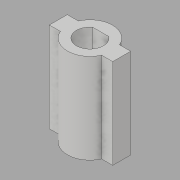
# Autodesk Inventor part: DispenserCoupling
Saved by Autodesk Inventor 2017 (Build 210142000, 142)
## iProperties
Created: 2017-02-22
Part Number: DispenserCoupling
Material: Generic
Document SubType Name: Modeling
Designer: gmarsh
Density: 1 g/cm^3
Appearance: Default
Author: gmarsh
Autodesk Inventor part; units mm, degrees
ref_plane "YZ Plane" through (0, 0, 0) normal (1, 0, 0) x (0, 1, 0)
ref_plane "XZ Plane" through (0, 0, 0) normal (0, 1, 0) x (-1, 0, 0)
ref_plane "XY Plane" through (0, 0, 0) normal (0, 0, 1) x (1, 0, 0)
sketch "Sketch1" plane through (0, 0, 0) normal (0, 0, 1) x (1, 0, 0)
  line L0 (7.0628, 2) -> (7.0628, -2)
  line L1 (-7.0394, -2) -> (-7.0394, 2)
  line L2 (-7.0394, 2) -> (-4.5826, 2)
  line L3 (4.5826, 2) -> (7.0628, 2)
  line L4 (7.0628, -2) -> (4.5826, -2)
  line L5 (-4.5826, -2) -> (-7.0394, -2)
  arc A0 (-4.5826, -2) -> (4.5826, -2) centre (0, 0) ccw
  arc A1 (4.5826, 2) -> (-4.5826, 2) centre (0, 0) ccw
  constraints: 12 end point, 5 parallel, 4 point on circle, 2 centre point, 2 horizontal, 2 perpendicular, 1 coincident
extrude "Extrusion1" add sketch "Sketch1" along normal blind 20
sketch "Sketch2" plane through (0, 0, 20) normal (0, 0, 1) x (1, 0, 0)
  arc A0 (-1.8, 2.4) -> (1.8, 2.4) centre (0, 0) ccw
  line L0 (-1.8, 2.4) -> (1.8, 2.4)
  dimension "d2" = 6
  constraints: 2 end point, 2 point on circle, 1 centre point, 1 coincident, 1 horizontal
  measures "d2" diameter of A0
extrude "Extrusion2" cut sketch "Sketch2" against normal blind 9
sketch "Sketch3" plane through (0, 0, 0) normal (0, 0, -1) x (-1, 0, 0)
  line L0 (2, 2) -> (-2, 2)
  line L1 (-2, 2) -> (-2, -2)
  line L2 (-2, -2) -> (2, -2)
  line L3 (2, -2) -> (2, 2)
  line L4 (2, 2) -> (-2, -2) construction
  line L5 (-2, 2) -> (2, -2) construction
  point P0 (0, 0)
  dimension "d5" = 4
  dimension "d6" = 4
  constraints: 12 end point, 2 midpoint, 2 parallel, 1 horizontal, 1 perpendicular
  measures "d5" distance of L2.end L1.end
  measures "d6" distance of L1.end L0.end
extrude "Extrusion3" cut sketch "Sketch3" against normal blind 9
body "Solid1"
